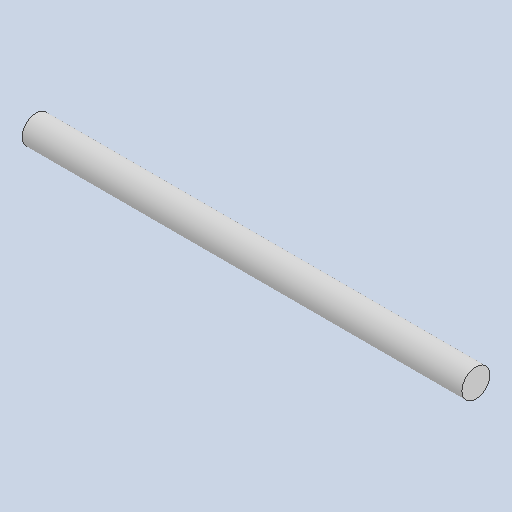
# Autodesk Inventor part: Вал движения головы
Saved by Autodesk Inventor 2023.2 (Build 272271030, 271C)
## iProperties
Created: 2024-02-18
Part Number: Вал движения головы
Material: Типовые
Document SubType Name: Modeling
Designer: I9232
Density: 1 g/cm^3
Appearance: По умолчанию
Author: I9232
Autodesk Inventor part; units mm, degrees
ref_plane "YZ Plane" through (0, 0, 0) normal (1, 0, 0) x (0, 1, 0)
ref_plane "XZ Plane" through (0, 0, 0) normal (0, 1, 0) x (-1, 0, 0)
ref_plane "XY Plane" through (0, 0, 0) normal (0, 0, 1) x (1, 0, 0)
sketch "Эскиз1" plane through (0, 0, 0) normal (0, 1, 0) x (-1, 0, 0)
  line L0 (-78.318, 0) -> (-78.318, -5)
  line L1 (-78.318, -5) -> (0, -5)
  line L2 (0, -21.8023) -> (0, 10.3406) construction
  line L3 (78.318, 0) -> (78.318, -5)
  line L4 (78.318, -5) -> (0, -5)
  line L5 (8.4814, 0) -> (-19.0918, 0) construction
  line L6 (78.318, 0) -> (-78.318, 0)
  point P0 (0, 0)
  dimension "d0" = 78.318
  dimension "d1" = 5
  constraints: 14 end point, 2 horizontal, 2 symmetric about line, 1 vertical
  measures "d0" distance of L0.end L1.end
  measures "d1" distance of L0.start L0.end
revolve "Вращение1" add sketch "Эскиз1" angle 360 about axis through (-8.4814, 0, 0) along (1, 0, 0)
